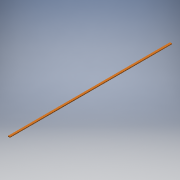
# Autodesk Inventor part: Lec30x70
Saved by Autodesk Inventor 2019 (Build 230136000, 136)
## iProperties
Created: 2022-04-03
Part Number: Lec30x70
Material: Gold
Document SubType Name: Modeling
Designer: laca
Mass: 243180 g
Surface Area: 12042 cm^2
Volume: 12600 cm^3
Density: 19.3 g/cm^3
Appearance: Metal 1600F Hot
Author: laca
Autodesk Inventor part; units mm, degrees
ref_plane "YZ Plane" through (0, 0, 0) normal (1, 0, 0) x (0, 1, 0)
ref_plane "XZ Plane" through (0, 0, 0) normal (0, 1, 0) x (-1, 0, 0)
ref_plane "XY Plane" through (0, 0, 0) normal (0, 0, 1) x (1, 0, 0)
sketch "Sketch1" plane through (0, 0, 0) normal (0, 0, 1) x (1, 0, 0)
  line L0 (0, 0) -> (-70, 0)
  line L1 (-70, 0) -> (-70, 30)
  line L2 (-70, 30) -> (0, 30)
  line L3 (0, 30) -> (0, 0)
  dimension "d0" = 70
  dimension "d1" = 30
  constraints: 8 end point, 2 parallel, 1 horizontal, 1 perpendicular
  measures "d0" distance of L1.end L2.end
  measures "d1" distance of L0.end L1.end
extrude "Extrusion1" add sketch "Sketch1" along normal blind 6000
body "Solid1"
